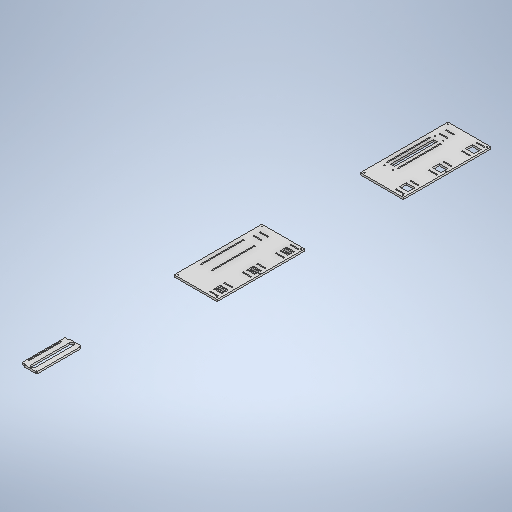
# Autodesk Inventor part: MODIFIED_CHASSIS
Saved by Autodesk Inventor 2025 (Build 290162000, 162)
## iProperties
Created: 2024-11-09
Part Number: MODIFIED_CHASSIS
Material: Generic
Document SubType Name: Modeling
Designer: Student
Density: 1 g/cm^3
Appearance: Default
Author: Student
Autodesk Inventor part; units mm, degrees
ref_plane "YZ Plane" through (0, 0, 0) normal (1, 0, 0) x (0, 1, 0)
ref_plane "XZ Plane" through (0, 0, 0) normal (0, 1, 0) x (-1, 0, 0)
ref_plane "XY Plane" through (0, 0, 0) normal (0, 0, 1) x (1, 0, 0)
sketch "Sketch1" plane through (0, 0, 0) normal (0, 1, 0) x (-1, 0, 0)
  line L0 (-199.6271, -109.7553) -> (0.3729, -109.7553)
  line L1 (0.3729, -559.7553) -> (-199.6271, -559.7553)
  line L2 (-199.6271, -559.7553) -> (-199.6271, -109.7553)
  line L3 (-184.6271, -369.7553) -> (-144.6271, -369.7553)
  line L4 (-144.6271, -369.7553) -> (-144.6271, -374.7553)
  line L5 (-144.6271, -374.7553) -> (-184.6271, -374.7553)
  line L6 (-184.6271, -374.7553) -> (-184.6271, -369.7553)
  line L7 (-184.6271, -369.7553) -> (-144.6271, -374.7553) construction
  line L8 (-144.6271, -369.7553) -> (-184.6271, -374.7553) construction
  line L9 (-184.6271, -299.7553) -> (-144.6271, -299.7553)
  line L10 (-144.6271, -299.7553) -> (-144.6271, -294.7553)
  line L11 (-144.6271, -294.7553) -> (-184.6271, -294.7553)
  line L12 (-184.6271, -294.7553) -> (-184.6271, -299.7553)
  line L13 (-187.1271, -146.7553) -> (-142.1271, -146.7553)
  line L14 (-142.1271, -146.7553) -> (-142.1271, -182.7553)
  line L15 (-142.1271, -182.7553) -> (-187.1271, -182.7553)
  line L16 (-187.1271, -182.7553) -> (-187.1271, -146.7553)
  line L17 (-187.1271, -146.7553) -> (-142.1271, -182.7553) construction
  line L18 (-142.1271, -146.7553) -> (-187.1271, -182.7553) construction
  line L19 (-142.1271, -486.7553) -> (-187.1271, -486.7553)
  line L20 (-187.1271, -486.7553) -> (-187.1271, -522.7553)
  line L21 (-187.1271, -522.7553) -> (-142.1271, -522.7553)
  line L22 (-187.1271, -522.7553) -> (-142.1271, -486.7553) construction
  line L23 (-142.1271, -522.7553) -> (-187.1271, -486.7553) construction
  line L24 (-142.1271, -522.7553) -> (-142.1271, -486.7553)
  line L25 (-187.1271, -316.7553) -> (-142.1271, -316.7553)
  line L26 (-142.1271, -316.7553) -> (-142.1271, -352.7553)
  line L27 (-142.1271, -352.7553) -> (-187.1271, -352.7553)
  line L28 (-187.1271, -352.7553) -> (-187.1271, -316.7553)
  line L29 (-187.1271, -316.7553) -> (-142.1271, -352.7553) construction
  line L30 (-142.1271, -316.7553) -> (-187.1271, -352.7553) construction
  line L31 (-49.6271, -484.7553) -> (-9.6271, -484.7553)
  line L32 (-9.6271, -484.7553) -> (-9.6271, -489.7553)
  line L33 (-9.6271, -489.7553) -> (-49.6271, -489.7553)
  line L34 (-49.6271, -489.7553) -> (-49.6271, -484.7553)
  line L35 (-49.6271, -484.7553) -> (-9.6271, -489.7553) construction
  line L36 (-9.6271, -484.7553) -> (-49.6271, -489.7553) construction
  line L37 (-49.6271, -516.7553) -> (-9.6271, -516.7553)
  line L38 (-9.6271, -516.7553) -> (-9.6271, -521.7553)
  line L39 (-9.6271, -521.7553) -> (-49.6271, -521.7553)
  line L40 (-49.6271, -521.7553) -> (-49.6271, -516.7553)
  line L41 (-49.6271, -516.7553) -> (-9.6271, -521.7553) construction
  line L42 (-9.6271, -516.7553) -> (-49.6271, -521.7553) construction
  line L43 (-39.6271, -224.7553) -> (-19.6271, -224.7553)
  line L44 (-19.6271, -224.7553) -> (-19.6271, -444.7553)
  line L45 (-19.6271, -444.7553) -> (-39.6271, -444.7553)
  line L46 (-39.6271, -444.7553) -> (-39.6271, -224.7553)
  line L47 (-39.6271, -224.7553) -> (-19.6271, -444.7553) construction
  line L48 (-19.6271, -224.7553) -> (-39.6271, -444.7553) construction
  line L49 (0.3729, -109.7553) -> (-19.6271, -109.7553)
  circle A0 centre (-189.6271, -119.7553) radius 3
  circle A1 centre (-189.6271, -549.7553) radius 3
  circle A2 centre (-193.6271, -334.7553) radius 3
  line L50 (-175.7177, 822.9635) -> (24.2823, 822.9635)
  line L51 (-160.7177, 562.9635) -> (-120.7177, 562.9635)
  line L52 (-160.7177, 557.9635) -> (-160.7177, 562.9635)
  line L53 (-120.7177, 557.9635) -> (-160.7177, 557.9635)
  line L54 (-120.7177, 562.9635) -> (-120.7177, 557.9635)
  line L55 (-120.7177, 562.9635) -> (-160.7177, 557.9635) construction
  line L56 (-160.7177, 562.9635) -> (-120.7177, 557.9635) construction
  line L57 (-175.7177, 372.9635) -> (-175.7177, 822.9635)
  line L58 (24.2823, 372.9635) -> (-175.7177, 372.9635)
  line L59 (24.2823, 822.9635) -> (4.2823, 822.9635)
  circle A3 centre (-169.7177, 597.9635) radius 3
  line L60 (-25.7177, 410.9635) -> (-25.7177, 415.9635)
  line L61 (-25.7177, 442.9635) -> (-25.7177, 447.9635)
  line L62 (14.2823, 415.9635) -> (14.2823, 410.9635)
  line L63 (-25.7177, 415.9635) -> (14.2823, 410.9635) construction
  line L64 (14.2823, 415.9635) -> (-25.7177, 410.9635) construction
  line L65 (14.2823, 410.9635) -> (-25.7177, 410.9635)
  line L66 (-25.7177, 415.9635) -> (14.2823, 415.9635)
  line L67 (14.2823, 442.9635) -> (-25.7177, 442.9635)
  line L68 (-25.7177, 447.9635) -> (14.2823, 447.9635)
  line L69 (14.2823, 447.9635) -> (14.2823, 442.9635)
  line L70 (-25.7177, 447.9635) -> (14.2823, 442.9635) construction
  line L71 (14.2823, 447.9635) -> (-25.7177, 442.9635) construction
  circle A4 centre (-165.7177, 812.9635) radius 3
  line L72 (-160.7177, 732.9635) -> (-120.7177, 732.9635)
  line L73 (-120.7177, 727.9635) -> (-160.7177, 727.9635)
  line L74 (-160.7177, 727.9635) -> (-160.7177, 732.9635)
  line L75 (-160.7177, 732.9635) -> (-120.7177, 727.9635) construction
  line L76 (-120.7177, 732.9635) -> (-160.7177, 727.9635) construction
  line L77 (-120.7177, 732.9635) -> (-120.7177, 727.9635)
  circle A5 centre (-165.7177, 382.9635) radius 3
  line L78 (-160.7177, 761.9635) -> (-120.7177, 761.9635)
  line L79 (-120.7177, 761.9635) -> (-120.7177, 773.9635)
  line L80 (-120.7177, 773.9635) -> (-160.7177, 773.9635)
  line L81 (-160.7177, 773.9635) -> (-160.7177, 761.9635)
  line L82 (-160.7177, 761.9635) -> (-120.7177, 773.9635) construction
  line L83 (-120.7177, 761.9635) -> (-160.7177, 773.9635) construction
  line L84 (-160.7177, 603.9635) -> (-120.7177, 603.9635)
  line L85 (-120.7177, 603.9635) -> (-120.7177, 591.9635)
  line L86 (-120.7177, 591.9635) -> (-160.7177, 591.9635)
  line L87 (-160.7177, 591.9635) -> (-160.7177, 603.9635)
  line L88 (-160.7177, 603.9635) -> (-120.7177, 591.9635) construction
  line L89 (-120.7177, 603.9635) -> (-160.7177, 591.9635) construction
  line L90 (-120.7177, 433.9635) -> (-120.7177, 421.9635)
  line L91 (-120.7177, 421.9635) -> (-160.7177, 421.9635)
  line L92 (-160.7177, 421.9635) -> (-160.7177, 433.9635)
  line L93 (-160.7177, 433.9635) -> (-120.7177, 421.9635) construction
  line L94 (-120.7177, 433.9635) -> (-160.7177, 421.9635) construction
  line L95 (-160.7177, 433.9635) -> (-120.7177, 433.9635)
  line L96 (-160.7177, 807.9635) -> (-120.7177, 807.9635)
  line L97 (-120.7177, 807.9635) -> (-120.7177, 802.9635)
  line L98 (-120.7177, 802.9635) -> (-160.7177, 802.9635)
  line L99 (-160.7177, 802.9635) -> (-160.7177, 807.9635)
  line L100 (-160.7177, 807.9635) -> (-120.7177, 802.9635) construction
  line L101 (-120.7177, 807.9635) -> (-160.7177, 802.9635) construction
  line L102 (-120.7177, 632.9635) -> (-120.7177, 637.9635)
  line L103 (-120.7177, 637.9635) -> (-160.7177, 637.9635)
  line L104 (-160.7177, 632.9635) -> (-120.7177, 632.9635)
  line L105 (-120.7177, 632.9635) -> (-160.7177, 637.9635) construction
  line L106 (-160.7177, 632.9635) -> (-120.7177, 637.9635) construction
  line L107 (-160.7177, 637.9635) -> (-160.7177, 632.9635)
  line L108 (-160.7177, 392.9635) -> (-160.7177, 387.9635)
  line L109 (-120.7177, 392.9635) -> (-160.7177, 392.9635)
  line L110 (-120.7177, 387.9635) -> (-120.7177, 392.9635)
  line L111 (-160.7177, 387.9635) -> (-120.7177, 392.9635) construction
  line L112 (-120.7177, 387.9635) -> (-160.7177, 392.9635) construction
  line L113 (-160.7177, 387.9635) -> (-120.7177, 387.9635)
  line L114 (-120.7177, 462.9635) -> (-120.7177, 467.9635)
  line L115 (-160.7177, 462.9635) -> (-120.7177, 462.9635)
  line L116 (-160.7177, 467.9635) -> (-160.7177, 462.9635)
  line L117 (-120.7177, 467.9635) -> (-160.7177, 467.9635)
  line L118 (-120.7177, 462.9635) -> (-160.7177, 467.9635) construction
  line L119 (-160.7177, 462.9635) -> (-120.7177, 467.9635) construction
  line L120 (-184.6271, -199.7553) -> (-144.6271, -199.7553)
  line L121 (-144.6271, -199.7553) -> (-144.6271, -204.7553)
  line L122 (-144.6271, -204.7553) -> (-184.6271, -204.7553)
  line L123 (-184.6271, -204.7553) -> (-184.6271, -199.7553)
  line L124 (-184.6271, -199.7553) -> (-144.6271, -204.7553) construction
  line L125 (-144.6271, -199.7553) -> (-184.6271, -204.7553) construction
  line L126 (-144.6271, -129.7553) -> (-144.6271, -124.7553)
  line L127 (-144.6271, -124.7553) -> (-184.6271, -124.7553)
  line L128 (-144.6271, -129.7553) -> (-184.6271, -124.7553) construction
  line L129 (-184.6271, -129.7553) -> (-144.6271, -124.7553) construction
  line L130 (-184.6271, -124.7553) -> (-184.6271, -129.7553)
  line L131 (-184.6271, -129.7553) -> (-144.6271, -129.7553)
  line L132 (-144.6271, -464.7553) -> (-184.6271, -464.7553)
  line L133 (-184.6271, -464.7553) -> (-184.6271, -469.7553)
  line L134 (-184.6271, -469.7553) -> (-144.6271, -464.7553) construction
  line L135 (-144.6271, -469.7553) -> (-184.6271, -464.7553) construction
  line L136 (-184.6271, -469.7553) -> (-144.6271, -469.7553)
  line L137 (-144.6271, -469.7553) -> (-144.6271, -464.7553)
  line L138 (-144.6271, -539.7553) -> (-144.6271, -544.7553)
  line L139 (-144.6271, -544.7553) -> (-184.6271, -544.7553)
  line L140 (-144.6271, -539.7553) -> (-184.6271, -544.7553) construction
  line L141 (-184.6271, -539.7553) -> (-144.6271, -544.7553) construction
  line L142 (-184.6271, -544.7553) -> (-184.6271, -539.7553)
  line L143 (-184.6271, -539.7553) -> (-144.6271, -539.7553)
  line L144 (-120.7177, 444.6635) -> (-160.7177, 444.6635)
  line L145 (-160.7177, 444.6635) -> (-160.7177, 439.6635)
  line L146 (-160.7177, 439.6635) -> (-120.7177, 439.6635)
  line L147 (-120.7177, 439.6635) -> (-120.7177, 444.6635)
  line L148 (-120.7177, 444.6635) -> (-160.7177, 439.6635) construction
  line L149 (-160.7177, 444.6635) -> (-120.7177, 439.6635) construction
  line L150 (-160.7177, 416.2635) -> (-120.7177, 416.2635)
  line L151 (-160.7177, 411.2635) -> (-160.7177, 416.2635)
  line L152 (-120.7177, 411.2635) -> (-160.7177, 411.2635)
  line L153 (-120.7177, 411.2635) -> (-160.7177, 416.2635) construction
  line L154 (-160.7177, 411.2635) -> (-120.7177, 416.2635) construction
  line L155 (-120.7177, 416.2635) -> (-120.7177, 411.2635)
  line L156 (-120.7177, 581.2635) -> (-160.7177, 581.2635)
  line L157 (-160.7177, 581.2635) -> (-160.7177, 586.2635)
  line L158 (-160.7177, 586.2635) -> (-120.7177, 586.2635)
  line L159 (-120.7177, 586.2635) -> (-120.7177, 581.2635)
  line L160 (-120.7177, 581.2635) -> (-160.7177, 586.2635) construction
  line L161 (-160.7177, 581.2635) -> (-120.7177, 586.2635) construction
  line L162 (-160.7177, 609.6635) -> (-120.7177, 609.6635)
  line L163 (-120.7177, 614.6635) -> (-160.7177, 614.6635)
  line L164 (-120.7177, 609.6635) -> (-120.7177, 614.6635)
  line L165 (-120.7177, 614.6635) -> (-160.7177, 609.6635) construction
  line L166 (-160.7177, 614.6635) -> (-120.7177, 609.6635) construction
  line L167 (-160.7177, 614.6635) -> (-160.7177, 609.6635)
  line L168 (-140.7177, 597.9635) -> (-154.3563, 597.9635)
  line L169 (-160.7177, 779.6635) -> (-120.7177, 779.6635)
  line L170 (-120.7177, 784.6635) -> (-160.7177, 784.6635)
  line L171 (-120.7177, 784.6635) -> (-160.7177, 779.6635) construction
  line L172 (-160.7177, 784.6635) -> (-120.7177, 779.6635) construction
  line L173 (-120.7177, 779.6635) -> (-120.7177, 784.6635)
  line L174 (-160.7177, 784.6635) -> (-160.7177, 779.6635)
  line L175 (-120.7177, 756.2635) -> (-120.7177, 751.2635)
  line L176 (-160.7177, 756.2635) -> (-120.7177, 756.2635)
  line L177 (-160.7177, 751.2635) -> (-160.7177, 756.2635)
  line L178 (-120.7177, 751.2635) -> (-160.7177, 756.2635) construction
  line L179 (-160.7177, 751.2635) -> (-120.7177, 756.2635) construction
  line L180 (-120.7177, 751.2635) -> (-160.7177, 751.2635)
  line L181 (-54.6271, -224.7553) -> (-59.6271, -224.7553)
  line L182 (-59.6271, -224.7553) -> (-59.6271, -444.7553)
  line L183 (-59.6271, -444.7553) -> (-54.6271, -444.7553)
  line L184 (-54.6271, -444.7553) -> (-54.6271, -224.7553)
  line L185 (-54.6271, -224.7553) -> (-59.6271, -444.7553) construction
  line L186 (-59.6271, -224.7553) -> (-54.6271, -444.7553) construction
  circle A6 centre (-8.6271, -464.7553) radius 3
  circle A7 centre (-50.6271, -464.7553) radius 3
  circle A8 centre (-50.6271, -204.7553) radius 3
  circle A9 centre (-8.6271, -204.7553) radius 3
  line L187 (0.3729, -444.7553) -> (-4.6271, -444.7553)
  line L188 (0.3729, -224.7553) -> (0.3729, -444.7553)
  line L189 (-4.6271, -224.7553) -> (0.3729, -444.7553) construction
  line L190 (0.3729, -224.7553) -> (-4.6271, -444.7553) construction
  line L191 (-4.6271, -444.7553) -> (-4.6271, -224.7553)
  line L192 (-4.6271, -224.7553) -> (0.3729, -224.7553)
  line L193 (0.3729, -559.7553) -> (20.3729, -559.7553)
  line L194 (20.3729, -559.7553) -> (20.3729, -109.7553)
  line L195 (20.3729, -109.7553) -> (0.3729, -109.7553)
  circle A10 centre (10.3729, -119.7553) radius 3
  circle A11 centre (10.3729, -549.7553) radius 3
  line L196 (24.2823, 372.9635) -> (44.2823, 372.9635)
  line L197 (44.2823, 372.9635) -> (44.2823, 822.9635)
  line L198 (44.2823, 822.9635) -> (24.2823, 822.9635)
  circle A12 centre (34.2823, 382.9635) radius 3
  circle A13 centre (34.2823, 812.9635) radius 3
  line L199 (24.2823, 707.9635) -> (19.2823, 707.9635)
  line L200 (19.2823, 707.9635) -> (19.2823, 487.9635)
  line L201 (19.2823, 487.9635) -> (24.2823, 487.9635)
  line L202 (24.2823, 487.9635) -> (24.2823, 707.9635)
  line L203 (24.2823, 707.9635) -> (19.2823, 487.9635) construction
  line L204 (19.2823, 707.9635) -> (24.2823, 487.9635) construction
  line L205 (-35.7177, 707.9635) -> (-30.7177, 707.9635)
  line L206 (-30.7177, 707.9635) -> (-30.7177, 487.9635)
  line L207 (-30.7177, 487.9635) -> (-35.7177, 487.9635)
  line L208 (-35.7177, 487.9635) -> (-35.7177, 707.9635)
  line L209 (-35.7177, 707.9635) -> (-30.7177, 487.9635) construction
  line L210 (-30.7177, 707.9635) -> (-35.7177, 487.9635) construction
  line L211 (-30, 1609.0073) -> (30, 1609.0073)
  line L212 (45, 1604.0073) -> (45, 1384.0073)
  line L213 (30, 1379.0073) -> (-30, 1379.0073)
  line L214 (-45, 1609.0073) -> (45, 1379.0073) construction
  line L215 (45, 1609.0073) -> (-45, 1379.0073) construction
  line L216 (30, 1379.0073) -> (30, 1384.0073)
  line L217 (30, 1384.0073) -> (45, 1384.0073)
  line L218 (30, 1609.0073) -> (30, 1604.0073)
  line L219 (30, 1604.0073) -> (45, 1604.0073)
  line L220 (0, 1379.0073) -> (-30, 1379.0073)
  line L221 (-30, 1379.0073) -> (-30, 1384.0073)
  line L222 (-30, 1384.0073) -> (-35, 1384.0073)
  line L223 (-30, 1609.0073) -> (-30, 1604.0073)
  line L224 (-30, 1604.0073) -> (-35, 1604.0073)
  line L225 (-35, 1604.0073) -> (-35, 1384.0073)
  line L226 (35, 1579.0073) -> (40, 1579.0073)
  line L227 (40, 1579.0073) -> (40, 1409.0073)
  line L228 (40, 1409.0073) -> (35, 1409.0073)
  line L229 (35, 1409.0073) -> (35, 1579.0073)
  line L230 (35, 1579.0073) -> (40, 1409.0073) construction
  line L231 (40, 1579.0073) -> (35, 1409.0073) construction
  line L232 (11, 1593.0073) -> (11, 1395.0073)
  line L233 (-11, 1395.0073) -> (-11, 1593.0073)
  line L234 (-11, 1604.0073) -> (11, 1384.0073) construction
  line L235 (11, 1604.0073) -> (-11, 1384.0073) construction
  arc A14 (11, 1593.0073) -> (-11, 1593.0073) centre (0, 1593.0073) ccw
  line L236 (-11, 1604.0073) -> (-9.6271, 1604.0073)
  line L237 (-4.6271, 1604.0073) -> (0, 1604.0073)
  arc A15 (-11, 1395.0073) -> (11, 1395.0073) centre (0, 1395.0073) ccw
  point P0 (0, 0)
  point P1 (-99.6271, -334.7553)
  point P2 (-75.7177, 597.9635)
  dimension "d0" = 200
  dimension "d1" = 40
  dimension "d2" = 5
  dimension "d3" = 220
  dimension "d4" = 200
  dimension "d5" = 40
  dimension "d6" = 5
  dimension "d7" = 12
  dimension "d8" = 40
  dimension "d9" = 5
  dimension "d10" = 40
  dimension "d11" = 5
  dimension "d12" = 36
  dimension "d13" = 45
  dimension "d14" = 5
  dimension "d15" = 5
  dimension "d16" = 5
  dimension "d17" = 220
  dimension "d18" = 20
  dimension "d19" = 450
  dimension "d20" = 20
  dimension "d21" = 450
  dimension "d22" = 5
  dimension "d23" = 220
  dimension "d24" = 5
  dimension "d25" = 90
  dimension "d26" = 230
  dimension "d28" = 5
  dimension "d29" = 30
  dimension "d30" = 5
  dimension "d31" = 5
  dimension "d33" = 5
  dimension "d34" = 170
  dimension "d35" = 22
  dimension "d36" = 220
  constraints: 476 end point, 44 parallel, 31 horizontal, 25 perpendicular, 16 centre point, 8 symmetric about line, 5 point on circle, 2 midpoint, 2 point on line, 1 tangent, 1 vertical
  measures "d0" distance of L1.start L1.end
  measures "d1" distance of L32.end L34.start
  measures "d2" distance of L31.end L32.end
  measures "d3" distance of L43.end L44.end
  measures "d4" distance of L196.start L57.start
  measures "d5" distance of L69.end L61.start
  measures "d6" distance of L69.start L69.end
  measures "d7" distance of L79.end L78.end
  measures "d8" distance of L86.start L86.end
  measures "d9" distance of L96.end L98.start
  measures "d10" distance of L122.start L122.end
  measures "d11" distance of L120.end L122.start
  measures "d12" distance of L15.end L13.start
  measures "d13" distance of L13.start L13.end
  measures "d14" distance of L146.start L144.end
  measures "d15" distance of L156.end L160.end
  measures "d16" distance of L184.start L182.end
  measures "d17" distance between parallel lines of L181 L183
  measures "d18" distance of L1.start L194.start
  measures "d19" distance of L194.start L194.end
  measures "d20" distance of L196.start L197.start
  measures "d21" distance of L197.start L197.end
  measures "d22" distance of L204.end L200.end
  measures "d23" distance of L200.end L199.end
  measures "d24" distance of L207.start L207.end
  measures "d25" distance of L214.end L215.end
  measures "d26" distance of L215.start L214.end
  measures "d28" distance of L213.start L216.end
  measures "d29" distance of L213.end L220.start
  measures "d30" distance of L213.end L221.end
  measures "d31" distance of L221.end L222.end
  measures "d33" distance of L227.end L228.end
  measures "d34" distance of L226.end L227.end
  measures "d35" distance of L234.end L235.end
  measures "d36" distance of L235.start L234.end
extrude "Extrusion1" add sketch "Sketch1" along normal blind 10
body "Solid1"
